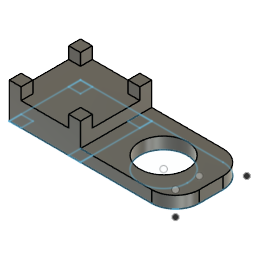
Ex5-lab1 (Autodesk Fusion 360 design; units mm, degrees)
part number: 2026-03-04-00-22-08-428
Autodesk Fusion 360 part; units mm, degrees
sketch "Sketch1" plane through (0, 0, 0) normal (0, 0, 1) x (1, 0, 0)
  line L0 (62.7035, 16.041) -> (62.7035, 166.041)
  line L1 (62.7035, 16.041) -> (362.7035, 16.041)
  line L2 (62.7035, 166.041) -> (362.7035, 166.041)
  line L3 (412.7035, 116.041) -> (412.7035, 66.041)
  arc A0 (412.7035, 116.041) -> (362.7035, 166.041) centre (362.7035, 116.041) ccw
  arc A1 (362.7035, 16.041) -> (412.7035, 66.041) centre (362.7035, 66.041) ccw
  line L4 (212.7035, 166.041) -> (212.7035, 16.041)
  circle A2 centre (312.7035, 91.041) radius 50
  line L5 (62.7035, 166.041) -> (87.7035, 166.041)
  line L6 (87.7035, 166.041) -> (87.7035, 141.041)
  line L7 (87.7035, 141.041) -> (62.7035, 141.041)
  line L8 (62.7035, 141.041) -> (62.7035, 166.041)
  line L9 (212.7035, 166.041) -> (187.7035, 166.041)
  line L10 (187.7035, 166.041) -> (187.7035, 141.041)
  line L11 (187.7035, 141.041) -> (212.7035, 141.041)
  line L12 (212.7035, 141.041) -> (212.7035, 166.041)
  line L13 (62.7035, 16.041) -> (87.7035, 16.041)
  line L14 (87.7035, 16.041) -> (87.7035, 41.041)
  line L15 (87.7035, 41.041) -> (62.7035, 41.041)
  line L16 (62.7035, 41.041) -> (62.7035, 16.041)
  line L17 (212.7035, 16.041) -> (187.7035, 16.041)
  line L18 (187.7035, 16.041) -> (187.7035, 41.041)
  line L19 (187.7035, 41.041) -> (212.7035, 41.041)
  line L20 (212.7035, 41.041) -> (212.7035, 16.041)
  point P0 (412.7035, 16.041)
  point P1 (412.7035, 166.041)
  dimension "d1" = 150
  dimension "d2" = 350
  dimension "d3" = 350
  dimension "d4" = 50
  dimension "d5" = 50
  dimension "d8" = 100
  dimension "d9" = 25
  dimension "d10" = 25
  dimension "d11" = 25
  dimension "d12" = 25
  dimension "d13" = 25
  dimension "d14" = 25
  dimension "d15" = 25
  dimension "d16" = 25
  constraint vertical L0
  constraint perpendicular L0 L1
  constraint perpendicular L0 L2
  constraint coincident P1 L2
  constraint coincident P1 L3
  constraint tangent L2 A0
  constraint tangent L3 A0
  constraint coincident P0 L1
  constraint coincident P0 L3
  constraint tangent L1 A1
  constraint tangent L3 A1
  constraint midpoint L1 L4.end
  constraint horizontal L5
  constraint vertical L6
  constraint horizontal L7
  constraint vertical L8
  constraint horizontal L9
  constraint vertical L10
  constraint horizontal L11
  constraint vertical L12
  constraint horizontal L13
  constraint vertical L14
  constraint horizontal L15
  constraint vertical L16
  constraint horizontal L17
  constraint vertical L18
  constraint horizontal L19
  constraint vertical L20
  measures "d1" distance of L0.start L0.end
  measures "d2" distance of L0.start P0
  measures "d3" distance of L0.end P1
  measures "d4" radius of A0
  measures "d5" radius of A1
  measures "d8" diameter of A2
  measures "d9" distance of L0.end L5.end
  measures "d10" distance of L0.end L7.end
  measures "d11" distance of L4.start L9.end
  measures "d12" distance of L4.start L11.end
  measures "d13" distance of L0.start L13.end
  measures "d14" distance of L0.start L15.end
  measures "d15" distance of L4.end L17.end
  measures "d16" distance of L4.end L19.end
extrude "Extrude1" add sketch "Sketch1" along normal blind 25 contours L1 L2 L3 A0 A1 L4 L12 L20
extrude "Extrude2" add sketch "Sketch1" along normal blind 50 contours L0 L1 L2 L4 L6 L7 L10 L11 L14 L15 L18 L19
extrude "Extrude3" add sketch "Sketch1" along normal blind 75 contours L0 L1 L13 L14 L15 L16 | L0 L2 L5 L6 L7 L8 | L1 L4 L17 L18 L19 L20 | L2 L4 L9 L10 L11 L12
